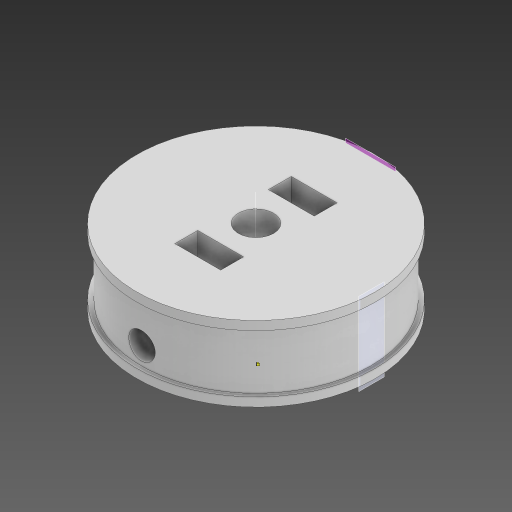
# Autodesk Inventor part: koleso
Saved by Autodesk Inventor 2023 (Build 270158000, 158)
## iProperties
Created: 2025-05-27
Part Number: koleso
Material: Типовые
Document SubType Name: Modeling
Designer: daa
Density: 1 g/cm^3
Appearance: По умолчанию
Author: daa
Autodesk Inventor part; units mm, degrees
ref_plane "YZ Plane" through (0, 0, 0) normal (1, 0, 0) x (0, 1, 0)
ref_plane "XZ Plane" through (0, 0, 0) normal (0, 1, 0) x (-1, 0, 0)
ref_plane "XY Plane" through (0, 0, 0) normal (0, 0, 1) x (1, 0, 0)
sketch "Эскиз1" plane through (0, 0, 0) normal (0, 1, 0) x (-1, 0, 0)
  circle A0 centre (0, 0) radius 13
  circle A1 centre (0, 0) radius 2
  dimension "d0" = 26
  dimension "d3" = 4
  constraints: 2 centre point, 2 coincident
  measures "d0" diameter of A0
  measures "d3" diameter of A1
extrude "Выдавливание1" add sketch "Эскиз1" along normal blind 6.5
sketch "Эскиз2" plane through (0, 6.5, 0) normal (0, 1, 0) x (1, 0, 0)
  circle A0 centre (0, 0) radius 13.5
  dimension "d4" = 27
  constraints: 1 centre point
  measures "d4" diameter of A0
extrude "Выдавливание2" add sketch "Эскиз2" along normal blind 1
sketch "Эскиз3" plane through (0, 0, 0) normal (0, -1, 0) x (1, 0, 0)
  circle A0 centre (0, 0) radius 13.5
  dimension "d7" = 27
  constraints: 1 centre point
  measures "d7" diameter of A0
extrude "Выдавливание3" add sketch "Эскиз3" along normal blind 1
sketch "Эскиз4" plane through (0, 7.5, 0) normal (0, 1, 0) x (1, 0, 0)
  circle A0 centre (0, 0) radius 2
  line L0 (2.6, -6.6) -> (-2.6, -6.6)
  line L1 (-2.6, -6.6) -> (-2.6, -4)
  line L2 (-2.6, -4) -> (2.6, -4)
  line L3 (2.6, -4) -> (2.6, -6.6)
  line L4 (2.6, 4) -> (-2.6, 4)
  line L5 (-2.6, 4) -> (-2.6, 6.6)
  line L6 (-2.6, 6.6) -> (2.6, 6.6)
  line L7 (2.6, 6.6) -> (2.6, 4)
  dimension "d12" = 4
  dimension "d13" = 5.2
  dimension "d14" = 2.6
  dimension "d15" = 2.6
  dimension "d16" = 4
  dimension "d17" = 5.2
  dimension "d18" = 2.6
  dimension "d19" = 2.6
  dimension "d20" = 4
  constraints: 16 end point, 4 parallel, 2 horizontal, 2 perpendicular, 1 centre point, 1 coincident
  measures "d12" diameter of A0
  measures "d13" distance of L1.end L2.end
  measures "d14" distance of L0.end L1.end
  measures "d15" distance from line of point (0, 0) L1
  measures "d16" distance from line of L2 point (0, 0)
  measures "d17" distance of L5.end L6.end
  measures "d18" distance of L4.end L5.end
  measures "d19" horizontal distance of L4.end point (0, 0)
  measures "d20" vertical distance of L4.end point (0, 0)
extrude "Выдавливание4" cut sketch "Эскиз4" against normal blind 8.75
ref_plane "РабПлоскость1" through (2.6, 7.5, -13) normal (0, 0, -1) x (-1, 0, 0)
sketch "Эскиз6" plane through (2.6, 7.5, -13) normal (0, 0, -1) x (-1, 0, 0)
  circle A0 centre (2.6, -5.5) radius 1.5
  line L0 (-10.9, -7.5) -> (16.1, -7.5) projected
  point P0 (2.6, -7.5)
  dimension "d24" = 3
  dimension "d25" = 2
  constraints: 1 centre point
  measures "d24" diameter of A0
  measures "d25" distance from line of L0 A0.centre
extrude "Выдавливание5" cut sketch "Эскиз6" against normal blind 27
ref_plane "РабПлоскость2" through (13.4, 7.5, -4) normal (1, 0, 0) x (0, 0, -1)
